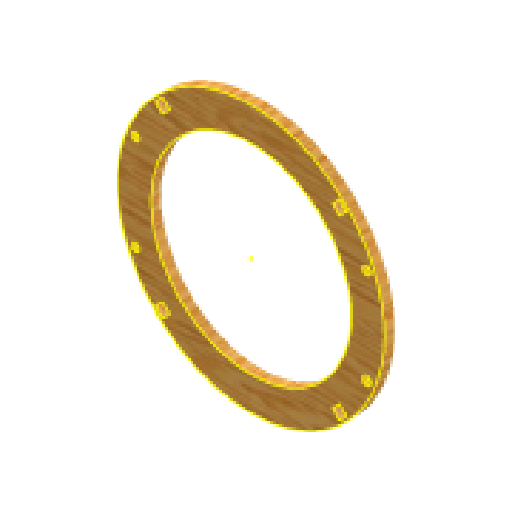
# Autodesk Inventor part: Front Ring New
Saved by Autodesk Inventor 2025.2 (Build 292293000, 293)
## iProperties
Created: 2025-01-15
Part Number: Front Ring New
Material: Plywood, Finish
Document SubType Name: Modeling
Designer: alexb
Density: 0.552 g/cm^3
Appearance: Plywood - New
Author: alexb
Autodesk Inventor part; units mm, degrees
ref_plane "YZ Plane" through (0, 0, 0) normal (1, 0, 0) x (0, 1, 0)
ref_plane "XZ Plane" through (0, 0, 0) normal (0, 1, 0) x (-1, 0, 0)
ref_plane "XY Plane" through (0, 0, 0) normal (0, 0, 1) x (1, 0, 0)
sketch "Sketch1" plane through (0, 0, 0) normal (0, 0, 1) x (1, 0, 0)
  circle A0 centre (0, 0) radius 80
  circle A1 centre (0, 0) radius 60
  circle A2 centre (0, 0) radius 70 construction
  line L0 (0, 0) -> (-60, 0)
  line L1 (0, 0) -> (-73.9104, 30.6147) construction
  circle A3 centre (-64.6716, 26.7878) radius 2.5
  circle A4 centre (-64.6716, -26.7878) radius 2.5
  line L2 (0, 0) -> (0, 60)
  line L3 (0, 0) -> (-56.5685, 56.5685) construction
  line L4 (-53.7401, 49.4975) -> (-49.4975, 45.2548)
  line L5 (-49.4975, 45.2548) -> (-45.2548, 49.4975)
  line L6 (-45.2548, 49.4975) -> (-49.4975, 53.7401)
  line L7 (-49.4975, 53.7401) -> (-53.7401, 49.4975)
  line L8 (-53.7401, 49.4975) -> (-45.2548, 49.4975) construction
  line L9 (-49.4975, 45.2548) -> (-49.4975, 53.7401) construction
  line L10 (-49.4975, -45.2548) -> (-53.7401, -49.4975)
  line L11 (-45.2548, -49.4975) -> (-49.4975, -45.2548)
  line L12 (-45.2548, -49.4975) -> (-53.7401, -49.4975) construction
  line L13 (-49.4975, -53.7401) -> (-49.4975, -45.2548) construction
  line L14 (-53.7401, -49.4975) -> (-49.4975, -53.7401)
  line L15 (-49.4975, -53.7401) -> (-45.2548, -49.4975)
  circle A5 centre (0, 0) radius 70 construction
  circle A6 centre (64.6716, 26.7878) radius 2.5
  circle A7 centre (64.6716, -26.7878) radius 2.5
  line L16 (53.7401, 49.4975) -> (49.4975, 45.2548)
  line L17 (49.4975, 45.2548) -> (45.2548, 49.4975)
  line L18 (45.2548, 49.4975) -> (49.4975, 53.7401)
  line L19 (49.4975, 53.7401) -> (53.7401, 49.4975)
  line L20 (53.7401, 49.4975) -> (45.2548, 49.4975) construction
  line L21 (49.4975, 45.2548) -> (49.4975, 53.7401) construction
  line L22 (49.4975, -45.2548) -> (53.7401, -49.4975)
  line L23 (45.2548, -49.4975) -> (49.4975, -45.2548)
  line L24 (45.2548, -49.4975) -> (53.7401, -49.4975) construction
  line L25 (49.4975, -53.7401) -> (49.4975, -45.2548) construction
  line L26 (53.7401, -49.4975) -> (49.4975, -53.7401)
  line L27 (49.4975, -53.7401) -> (45.2548, -49.4975)
  circle A8 centre (-69.291, 28.7013) radius 2.5
  circle A9 centre (-69.291, -28.7013) radius 2.5
  circle A10 centre (-28.7013, -69.291) radius 2.5
  circle A11 centre (28.7013, -69.291) radius 2.5
  circle A12 centre (69.291, -28.7013) radius 2.5
  circle A13 centre (69.291, 28.7013) radius 2.5
  circle A14 centre (28.7013, 69.291) radius 2.5
  circle A15 centre (-28.7013, 69.291) radius 2.5
  point P0 (-49.4975, 49.4975)
  point P1 (-49.4975, 49.4975)
  point P2 (-49.4975, 49.4975)
  point P3 (-49.4975, -49.4975)
  point P4 (-49.4975, -49.4975)
  point P5 (-49.4975, -49.4975)
  point P6 (49.4975, 49.4975)
  point P7 (49.4975, 49.4975)
  point P8 (49.4975, 49.4975)
  point P9 (49.4975, -49.4975)
  point P10 (49.4975, -49.4975)
  point P11 (49.4975, -49.4975)
  dimension "d4" = 140
  dimension "d6" = 22.5
  dimension "d7" = 5
  dimension "d8" = 160
  dimension "d11" = 45
  dimension "d13" = 20
  dimension "d16" = 45
  dimension "d19" = 6
  dimension "d20" = 6
  dimension "d23" = 90
  dimension "d27" = 5
  dimension "d28" = 75
  dimension "d31" = 360
  constraints: 56 end point, 16 centre point, 16 symmetric about line, 10 midpoint, 8 point on circle, 3 coincident, 3 point on line, 2 parallel, 2 perpendicular, 1 horizontal, 1 vertical, 37 other
  measures "d4" diameter of A2
  measures "d6" angle of L1 L0
  measures "d7" diameter of A3
  measures "d8" diameter of A0
  measures "d13" radial gap between concentric circles of A1 A0
  measures "d16" angle of L0 L3
  measures "d19" distance between parallel lines of L4 L6
  measures "d20" distance between parallel lines of L7 L5
  measures "d27" diameter of A8
  measures "d28" distance of point (0, 0) A8.centre
extrude "Extrusion1" add sketch "Sketch1" along normal blind 6 contours A0 | A3 | A4 | A6 | A7 | A10 | A11 | A14 | A15
equation "\"d20\" = d19"
body "Solid1"
